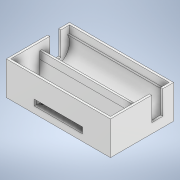
# Autodesk Inventor part: Bottom-Shell
Saved by Autodesk Inventor 2022 (Build 260153000, 153)
## iProperties
Company: El Camino College
Created: 2022-12-16
Part Number: Bottom-Shell
Material: ABS Plastic
Document SubType Name: Modeling
Designer: Edgar Tejada
Density: 1.06 g/cm^3
Appearance: Smooth - White
Project: Parametric-Modeling
Author: Edgar Tejada
Title: Battery Pack Bottom-Shell
Autodesk Inventor part; units mm, degrees
ref_plane "YZ Plane" through (0, 0, 0) normal (1, 0, 0) x (0, 1, 0)
ref_plane "XZ Plane" through (0, 0, 0) normal (0, 1, 0) x (-1, 0, 0)
ref_plane "XY Plane" through (0, 0, 0) normal (0, 0, 1) x (1, 0, 0)
sketch "Sketch1" plane through (0, 0, 0) normal (0, 1, 0) x (-1, 0, 0)
  line L0 (70, -42.5) -> (-70, -42.5)
  line L1 (-70, -42.5) -> (-70, 42.5)
  line L2 (-70, 42.5) -> (70, 42.5)
  line L3 (70, 42.5) -> (70, -42.5)
  line L4 (70, -42.5) -> (-70, 42.5) construction
  line L5 (-70, -42.5) -> (70, 42.5) construction
  point P0 (0, 0)
  dimension "d0" = 140
  dimension "d1" = 85
  constraints: 12 end point, 2 midpoint, 2 parallel, 1 horizontal, 1 perpendicular
  measures "d0" distance of L1.end L2.end
  measures "d1" distance of L2.end L0.start
extrude "Outer-Shell" add sketch "Sketch1" along normal blind 45
shell "Shell1" thickness 3 removed faces 1 at (-23.3333, 45, -14.1667)
sketch "Sketch2" plane through (-67, 3, 39.5) normal (0, 1, 0) x (1, 0, 0)
  line L0 (0, 79) -> (134, 79)
  line L1 (134, 79) -> (134, 39)
  line L2 (134, 39) -> (0, 39)
  line L3 (0, 39) -> (0, 79)
  line L4 (0, 79) -> (134, 39) construction
  line L5 (134, 79) -> (0, 39) construction
  line L6 (134, 0) -> (134, 79) projected
  line L7 (0, 79) -> (134, 79) projected
  line L8 (134, 79) -> (0, 79) projected
  line L9 (0, 79) -> (0, 0) projected
  point P0 (67, 39.5)
  point P1 (67, 59)
  dimension "d5" = 40
  constraints: 12 end point, 3 collinear, 2 midpoint, 2 parallel, 1 horizontal, 1 perpendicular
  measures "d5" distance of L2.end L0.start
extrude "Battery_Holder" add sketch "Sketch2" along normal blind 32
sketch "Sketch3" plane through (-67, 3, -39.5) normal (1, 0, 0) x (0, 0, -1)
  circle A0 centre (-20, 22) radius 20
  line L0 (-79, 42) -> (0, 42) projected
  line L1 (0, 0) -> (0, 42) projected
  point P0 (-39.5, -3)
  dimension "d8" = 40
  dimension "d9" = 20
  constraints: 1 centre point, 1 tangent
  measures "d8" diameter of A0
  measures "d9" distance from line of L0 A0.centre
extrude "Battery_Cutout" cut sketch "Sketch3" along normal up to surface (134 mm away) contours A0
sketch "Sketch4" plane through (-70, 0, -42.5) normal (-1, 0, 0) x (0, 0, 1)
  line L0 (14.5, 45) -> (29.5, 45)
  line L1 (29.5, 45) -> (29.5, 13)
  line L2 (29.5, 13) -> (14.5, 13)
  line L3 (14.5, 13) -> (14.5, 45)
  line L4 (0, 0) -> (0, 45) projected
  line L5 (0, 45) -> (85, 45) projected
  point P0 (42.5, 0)
  dimension "d15" = 15
  dimension "d16" = 32
  dimension "d17" = 14.5
  constraints: 8 end point, 2 parallel, 1 collinear, 1 horizontal, 1 perpendicular
  measures "d15" distance of L0.start L0.end
  measures "d16" distance of L0.end L1.end
  measures "d17" distance between parallel lines of L4 L3
extrude "Voltmeter_Cutouts" cut sketch "Sketch4" along normal through all both and the other way through all
sketch "Sketch5" plane through (0, 0, 0) normal (0, 1, 0) x (-1, 0, 0)
  line L0 (32, 10.5) -> (-32, 10.5)
  line L1 (-32, 10.5) -> (-32, 40.5)
  line L2 (-32, 40.5) -> (32, 40.5)
  line L3 (32, 40.5) -> (32, 10.5)
  line L4 (70, -13) -> (70, 42.5) projected
  line L5 (32, 40.5) -> (-32, 40.5)
  line L6 (-32, 40.5) -> (-32, 10.5)
  line L7 (-32, 10.5) -> (32, 10.5)
  line L8 (32, 10.5) -> (32, 40.5)
  line L9 (32, 40.5) -> (-32, 10.5) construction
  line L10 (-32, 40.5) -> (32, 10.5) construction
  point P0 (0, 0)
  point P1 (0, 25.5)
  point P2 (0, 25.5)
  dimension "d21" = 10.5
  dimension "d22" = 30
  dimension "d23" = 64
  constraints: 20 end point, 4 parallel, 3 midpoint, 2 collinear, 2 horizontal, 2 perpendicular, 1 vertical alignment
  measures "d21" distance from line of point (0, 0) L0
  measures "d22" distance of L0.end L1.end
  measures "d23" distance of L1.end L2.end
extrude "Controller_Stand" add sketch "Sketch5" along normal blind 9
sketch "Sketch6" plane through (-70, 0, 42.5) normal (0, 0, 1) x (1, 0, 0)
  line L0 (37.5, 17) -> (102.5, 17)
  line L1 (102.5, 17) -> (102.5, 9)
  line L2 (102.5, 9) -> (37.5, 9)
  line L3 (37.5, 9) -> (37.5, 17)
  line L4 (37.5, 17) -> (102.5, 9) construction
  line L5 (102.5, 17) -> (37.5, 9) construction
  line L6 (0, 0) -> (140, 0) projected
  point P0 (70, 0)
  point P1 (70, 13)
  dimension "d28" = 65
  dimension "d29" = 8
  dimension "d30" = 9
  constraints: 12 end point, 2 midpoint, 2 parallel, 1 horizontal, 1 perpendicular, 1 vertical alignment
  measures "d28" distance of L1.end L2.end
  measures "d29" distance of L2.end L0.start
  measures "d30" distance between parallel lines of L6 L2
extrude "USB_Access" cut sketch "Sketch6" against normal up to next
sketch "Sketch7" plane through (0, 0, 0) normal (0, 1, 0) x (-1, 0, 0)
  line L0 (29, 12) -> (-29, 12) construction
  line L1 (-29, 12) -> (-29, 35) construction
  line L2 (-29, 35) -> (29, 35) construction
  line L3 (29, 35) -> (29, 12) construction
  line L4 (29, 12) -> (-29, 35) construction
  line L5 (-29, 12) -> (29, 35) construction
  circle A0 centre (29, 12) radius 1.4
  circle A1 centre (-29, 12) radius 1.4
  circle A2 centre (-29, 35) radius 1.4
  circle A3 centre (29, 35) radius 1.4
  point P0 (0, 0)
  point P1 (0, 23.5)
  point P2 (0, 23.5)
  dimension "d33" = 23
  dimension "d34" = 58
  dimension "d35" = 12
  dimension "d36" = 2.8
  constraints: 12 end point, 4 centre point, 4 coincident, 3 equal radius, 3 midpoint, 2 parallel, 1 horizontal, 1 perpendicular, 1 vertical alignment
  measures "d33" distance of L0.end L1.end
  measures "d34" distance of L1.end L2.end
  measures "d35" distance from line of L0 point (0, 0)
  measures "d36" diameter of A0
extrude "M3_Mount_Holes" cut sketch "Sketch7" along normal through all both and the other way through all
equation "\"d1\" = 0.607143 * d0"
equation "\"d2\" = 0.321429 * d0"
equation "\"d4\" = 0.0214286 * d0"
equation "\"d5\" = 0.285714 * d0"
equation "\"d6\" = 0.8 * d5"
equation "\"d8\" = d5"
equation "\"d9\" = 0.142857 * d0"
equation "\"d10\" = d5"
equation "\"d15\" = 0.107143 * d0"
equation "\"d16\" = 0.228571 * d0"
equation "\"d17\" = 0.103571 * d0"
equation "\"d21\" = 0.075 * d0"
equation "\"d22\" = 0.214286 * d0"
equation "\"d23\" = 2.13333 * d22"
equation "\"d24\" = 0.3 * d22"
equation "\"d28\" = 2.16667 * d22"
equation "\"d29\" = 0.266667 * d22"
equation "\"d30\" = 0.3 * d22"
equation "\"d31\" = 0.3 * d22"
equation "\"d33\" = 0.164286 * d0"
equation "\"d34\" = 0.414286 * d0"
equation "\"d35\" = 0.0857143 * d0"
equation "\"d36\" = 0.02 * d0"
body "Solid1"
